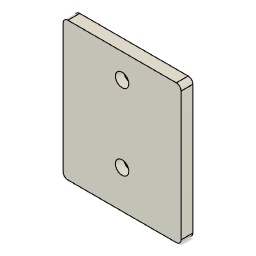
Battery_Spacer_v7 (Autodesk Fusion 360 design; units mm, degrees)
Autodesk Fusion 360 part; units mm, degrees
sketch "Sketch1" plane through (0, 0, 0) normal (0, 0, 1) x (1, 0, 0)
  line L0 (-12.45, 14.6) -> (12.45, 14.6)
  line L1 (12.45, 14.6) -> (12.45, -14.6)
  line L2 (12.45, -14.6) -> (-12.45, -14.6)
  line L3 (-12.45, -14.6) -> (-12.45, 14.6)
  line L4 (-12.45, -14.6) -> (12.45, 14.6) construction
  circle A0 centre (0, -6.6) radius 1.425
  circle A1 centre (0, -6.6) radius 2.75
  line L5 (0, 14.6) -> (0, -14.6) construction
  circle A2 centre (0, 9.4) radius 1.425
  circle A3 centre (0, 9.4) radius 2.75
  dimension "d1" = 24.9
  dimension "d2" = 29.2
  dimension "d92" = 2.85
  dimension "d98" = 5.5
  dimension "d141" = 8
  dimension "d142" = 16
  constraint horizontal L0
  constraint vertical L1
  constraint horizontal L2
  constraint vertical L3
  constraint midpoint origin L4
  constraint coincident A2.centre L5
  constraint concentric A2 A3
  constraint vertical L5
  constraint equal A0 A2
  constraint equal A1 A3
  constraint coincident A0.centre L5
  constraint coincident A0.centre A1.centre
  constraint coincident L2 L5.end
  constraint midpoint L0 L5.start
  measures "d1" distance of L0.start L0.end
  measures "d2" distance of L0.end L1.end
  measures "d92" diameter of A2
  measures "d98" diameter of A3
  measures "d141" distance of L5.end A0.centre
  measures "d142" distance of A2.centre A0.centre
extrude "Extrude1" add sketch "Sketch1" along normal blind 2.5 contours L0 L1 L2 L3 | A0 | A1 | A2 | A3
extrude "Extrude2" cut sketch "Sketch1" against normal blind 1.8 from surface at 2.5 contours A0 | A2
fillet "Fillet1" radius 1 4 edges at (-12.45, 14.6, 1.25) (12.45, 14.6, 1.25) (-12.45, -14.6, 1.25) (12.45, -14.6, 1.25)
